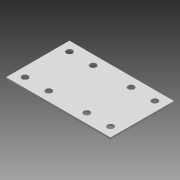
# Autodesk Inventor part: BracketUnfolded
Saved by Autodesk Inventor 2014 SP1 (Build 180222100, 222)
## iProperties
Created: 2015-03-22
Part Number: BracketUnfolded
Material: Generic
Document SubType Name: Sheet Metal
Designer: david
Density: 1 g/cm^3
Sheet Metal Rule: Default
Appearance: Default
Bracket_Hole_Diameter: 4,000 mm
Bracket_Holes_LateralDistance: 28,000 mm
Bracket_Holes_Distance: 15,000 mm
Bracket_Holes_UnfoldedDistance: 24,000 mm
Author: david
Autodesk Inventor part; units mm, degrees
ref_plane "YZ Plane" through (0, 0, 0) normal (1, 0, 0) x (0, 1, 0)
ref_plane "XZ Plane" through (0, 0, 0) normal (0, 1, 0) x (-1, 0, 0)
ref_plane "XY Plane" through (0, 0, 0) normal (0, 0, 1) x (1, 0, 0)
sketch "Sketch1" plane through (0, 0, 0) normal (0, 1, 0) x (-1, 0, 0)
  line L0 (-33, 20) -> (0, 20)
  line L1 (0, 20) -> (0, 0) construction
  line L2 (0, 0) -> (-33, 0) construction
  line L3 (-33, 0) -> (-33, 20)
  line L4 (-37.8717, 14) -> (4.6091, 14) construction
  circle A0 centre (-12, 14) radius 2
  circle A1 centre (-27, 14) radius 2
  line L5 (33, 20) -> (0, 20)
  line L6 (33, 0) -> (33, 20)
  line L7 (37.8717, 14) -> (-4.6091, 14) construction
  circle A2 centre (12, 14) radius 2
  circle A3 centre (27, 14) radius 2
  line L8 (-33, -20) -> (0, -20)
  line L9 (0, -20) -> (0, 0) construction
  line L10 (-33, 0) -> (-33, -20)
  line L11 (-37.8717, -14) -> (4.6091, -14) construction
  circle A4 centre (-12, -14) radius 2
  circle A5 centre (-27, -14) radius 2
  line L12 (33, -20) -> (0, -20)
  line L13 (37.8717, -14) -> (-4.6091, -14) construction
  circle A6 centre (12, -14) radius 2
  circle A7 centre (27, -14) radius 2
  line L14 (33, 0) -> (33, -20)
  dimension "d0" = 33
  dimension "d1" = 20
  dimension "d2" = 6
  dimension "Bracket_Hole_Diameter" = 4
  dimension "d4" = 6
  dimension "d5" = 21
  measures "d0" distance of L0.start L0.end
  measures "d1" distance of L2.end L0.start
  measures "d2" distance between parallel lines of L0 L4
  measures "Bracket_Hole_Diameter" diameter of A1
  measures "d4" distance from line of L3 A1.centre
  measures "d5" distance from line of L3 A0.centre
extrude "Plate1" add sketch "Sketch1" along normal blind 1
equation "\"BendRadius\" = Thickness"
equation "\"BendReliefWidth\" = Thickness"
equation "\"BendReliefDepth\" = 0.5 * Thickness"
equation "\"CornerReliefSize\" = 4 * Thickness"
equation "\"MinimumRemnant\" = 2 * Thickness"
equation "\"TransitionRadius\" = BendRadius"
equation "\"JacobiRadiusSize\" = BendRadius"
equation "\"GapSize\" = Thickness"
equation "\"d6\" = BendRadius"
equation "\"Bracket_Holes_LateralDistance\" = 28"
equation "\"Bracket_Holes_Distance\" = 15"
equation "\"Bracket_Holes_UnfoldedDistance\" = 24"
equation "\"Thickness\" = 1"
body "Solid1"
